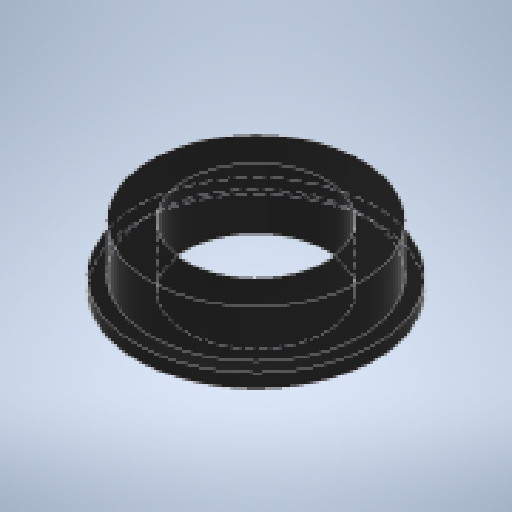
# Autodesk Inventor part: DDLF-1380zz
Saved by Autodesk Inventor 2025 (Build 290162000, 162)
## iProperties
Created: 2025-02-25
Part Number: DDLF-1380zz
Material: アセタール樹脂、黒
Document SubType Name: Modeling
Designer: Zhopa
Density: 1.425 g/cm^3
Appearance: 滑らか - 黒
Mass: 0.350048 g
Surface Area: 4.13936 cm^2
Volume: 0.245647 cm^3
Author: Zhopa
Autodesk Inventor part; units mm, degrees
ref_plane "YZ Plane" through (0, 0, 0) normal (1, 0, 0) x (0, 1, 0)
ref_plane "XZ Plane" through (0, 0, 0) normal (0, 1, 0) x (-1, 0, 0)
ref_plane "XY Plane" through (0, 0, 0) normal (0, 0, 1) x (1, 0, 0)
sketch "Sketch1" plane through (0, 0, 0) normal (1, 0, 0) x (0, 1, 0)
  line L0 (0, 0) -> (0, -6.8)
  line L1 (0, -6.8) -> (0.8, -6.8)
  line L2 (0.8, -6.8) -> (0.8, -6)
  line L3 (0.8, -6) -> (3.5, -6)
  line L4 (3.5, -6) -> (3.5, -4)
  line L5 (3.5, -4) -> (0, -4)
  line L6 (0, 0) -> (4.5024, 0)
  dimension "d0" = 6.8
  dimension "d1" = 0.8
  dimension "d2" = 0.8
  dimension "d3" = 2.7
  dimension "d4" = 2
  constraints: 14 end point, 4 perpendicular, 1 horizontal, 1 parallel, 1 point on line, 1 vertical
  measures "d0" distance of L0.start L0.end
  measures "d1" distance of L0.end L1.end
  measures "d2" distance of L1.end L2.end
  measures "d3" distance of L2.end L3.end
  measures "d4" distance of L3.end L4.end
revolve "Revolution1" add sketch "Sketch1" angle 360 about axis through (0, 0, 0) along (0, 1, 0)
body "Solid1"
